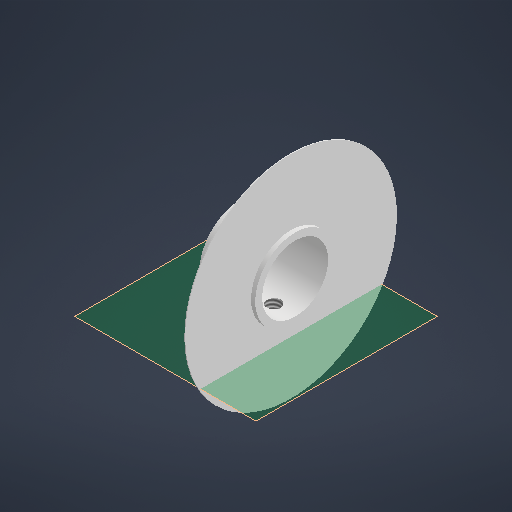
# Autodesk Inventor part: Tarcza impulsowa HEDS-5140
Saved by Autodesk Inventor 2026.1 (Build 301233020, 233B)
## iProperties
Created: 2026-03-26
Part Number: Tarcza impulsowa HEDS-5140
Material: Generic
Document SubType Name: Modeling
Designer: Jan
Density: 1 g/cm^3
Appearance: Default
Author: Jan
Autodesk Inventor part; units mm, degrees
ref_plane "YZ Plane" through (0, 0, 0) normal (1, 0, 0) x (0, 1, 0)
ref_plane "XZ Plane" through (0, 0, 0) normal (0, 1, 0) x (-1, 0, 0)
ref_plane "XY Plane" through (0, 0, 0) normal (0, 0, 1) x (1, 0, 0)
sketch "Sketch1" plane through (0, 0, 0) normal (0, 0, 1) x (1, 0, 0)
  line L0 (0, 0) -> (0, 5.08)
  line L1 (0, 5.08) -> (1.8, 5.08)
  line L2 (1.8, 5.08) -> (1.8, 6.35)
  line L3 (1.8, 6.35) -> (5.95, 6.35)
  line L4 (5.95, 6.35) -> (5.95, 12.85)
  line L5 (5.95, 12.85) -> (6.05, 12.85)
  line L6 (6.05, 12.85) -> (6.05, 4.85)
  line L7 (6.05, 4.85) -> (6.55, 4.85)
  line L8 (6.55, 4.85) -> (6.55, 0)
  line L9 (0, 0) -> (11.8727, 0) construction
  line L10 (0, 0) -> (6.55, 0)
  dimension "d0" = 5.08
  dimension "d1" = 1.8
  dimension "d2" = 1.27
  dimension "d3" = 4.15
  dimension "d4" = 6.5
  dimension "d5" = 0.1
  dimension "d6" = 8
  dimension "d7" = 0.5
  constraints: 22 end point, 7 perpendicular, 2 horizontal, 1 coincident, 1 collinear, 1 vertical
  measures "d0" distance of L0.start L0.end
  measures "d1" distance of L0.end L1.end
  measures "d2" distance of L1.end L2.end
  measures "d3" distance of L2.end L3.end
  measures "d4" distance of L3.end L4.end
  measures "d5" distance of L4.end L5.end
  measures "d6" distance of L5.end L6.end
  measures "d7" distance of L6.end L7.end
revolve "Revolution1" add sketch "Sketch1" angle 360 about axis through (0, 0, 0) along (1, 0, 0)
sketch "Sketch2" plane through (6.55, 0, 0) normal (1, 0, 0) x (0, 0, -1)
  circle A0 centre (0, 0) radius 4
  dimension "d9" = 8
  constraints: 1 centre point, 1 coincident
  measures "d9" diameter of A0
extrude "Extrusion1" cut sketch "Sketch2" against normal blind 10
sketch "Sketch3" plane through (1.8, 0, 0) normal (-1, 0, 0) x (0, 0, 1)
  circle A0 centre (0, 0) radius 6.35 projected
  point P0 (0, -6.35)
  constraints: 1 vertical alignment, 1 other
ref_plane "Work Plane1" through (1.8, -6.35, 0) normal (0, -1, 0) x (1, 0, 0)
sketch "Sketch4" plane through (1.8, -6.35, 0) normal (0, -1, 0) x (1, 0, 0)
  circle A0 centre (2.125, 0) radius 1.5
  line L0 (4.25, -12.85) -> (4.25, 12.85) projected
  line L1 (0, -6.35) -> (0, 6.35) projected
  point P0 (-1.8, 0)
  dimension "d12" = 3
  dimension "d14" = 4.25
  dimension "d15" = 2.125
  constraints: 1 centre point
  measures "d12" diameter of A0
  measures "d14" distance between parallel lines of L0 L1
  measures "d15" distance from line of L1 A0.centre
hole "Hole1" at (3.925, -6.35, 0) direction (0, 1, 0) diameter 1.6942 depth 6.637 tip angle 118 thread size "2-56 UNC" class "2B" standard "ANSI Unified Screw Threads"
equation "\"d15\" = 0.5 * d14"
body "Solid1"
